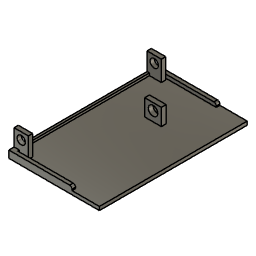
uselessbox-top-2 (Autodesk Fusion 360 design; units mm, degrees)
Autodesk Fusion 360 part; units mm, degrees
sketch "Sketch1" plane through (0, 0, 0) normal (0, 0, 1) x (1, 0, 0)
  line L0 (-25, 50) -> (13, 50)
  line L1 (13, 50) -> (13, -12)
  line L2 (13, -12) -> (-25, -12)
  line L3 (-25, -12) -> (-25, 50)
  line L4 (-25, 50) -> (-22.8, 50)
  line L5 (-22.8, 50) -> (-22.8, 47.8)
  line L6 (-22.8, 47.8) -> (-25, 47.8)
  line L7 (-25, 47.8) -> (-25, 50)
  line L8 (-25, 47.8) -> (-20, 47.8)
  line L9 (-20, 47.8) -> (-20, 47)
  line L10 (-20, 47) -> (-25, 47)
  line L11 (-25, 47) -> (-25, 47.8)
  line L12 (-25, -12) -> (-22.8, -12)
  line L13 (-22.8, -12) -> (-22.8, -9.8)
  line L14 (-22.8, -9.8) -> (-25, -9.8)
  line L15 (-25, -9.8) -> (-25, -12)
  line L16 (-25, -9.8) -> (-20, -9.8)
  line L17 (-20, -9.8) -> (-20, -9)
  line L18 (-20, -9) -> (-25, -9)
  line L19 (-25, -9) -> (-25, -9.8)
  line L20 (-25, -12) -> (3, -12)
  line L21 (3, -12) -> (3, -10.5)
  line L22 (3, -10.5) -> (-25, -10.5)
  line L23 (-25, -10.5) -> (-25, -12)
  line L24 (-25, 50) -> (3, 50)
  line L25 (3, 50) -> (3, 48.5)
  line L26 (3, 48.5) -> (-25, 48.5)
  line L27 (-25, 48.5) -> (-25, 50)
  dimension "d1" = 38
  dimension "d2" = 62
  dimension "d3" = 2.2
  dimension "d4" = 2.2
  dimension "d5" = 5
  dimension "d6" = 0.8
  dimension "d7" = 2.2
  dimension "d8" = 2.2
  dimension "d9" = 5
  dimension "d10" = 0.8
  dimension "d11" = 28
  dimension "d12" = 1.5
  dimension "d13" = 28
  dimension "d14" = 1.5
  constraint horizontal L0
  constraint vertical L1
  constraint horizontal L2
  constraint vertical L3
  constraint horizontal L4
  constraint vertical L5
  constraint horizontal L6
  constraint vertical L7
  constraint horizontal L8
  constraint vertical L9
  constraint horizontal L10
  constraint vertical L11
  constraint horizontal L12
  constraint vertical L13
  constraint horizontal L14
  constraint vertical L15
  constraint horizontal L16
  constraint vertical L17
  constraint horizontal L18
  constraint vertical L19
  constraint horizontal L20
  constraint vertical L21
  constraint horizontal L22
  constraint vertical L23
  constraint horizontal L24
  constraint vertical L25
  constraint horizontal L26
  constraint vertical L27
  measures "d1" distance of L0.start L0.end
  measures "d2" distance of L0.start L2.end
  measures "d3" distance of L0.start L4.end
  measures "d4" distance of L0.start L6.end
  measures "d5" distance of L6.end L8.end
  measures "d6" distance of L6.end L10.end
  measures "d7" distance of L2.end L12.end
  measures "d8" distance of L2.end L14.end
  measures "d9" distance of L14.end L16.end
  measures "d10" distance of L14.end L18.end
  measures "d11" distance of L2.end L20.end
  measures "d12" distance of L2.end L22.end
  measures "d13" distance of L0.start L24.end
  measures "d14" distance of L0.start L26.end
extrude "Extrude1" add sketch "Sketch1" along normal blind 6 contours L3 L6 L8 L9 L10 L11 | L3 L14 L16 L17 L18 L19 makes body 1 at (-21.6667, 47.8, 2) makes body 2 at (-21.6667, -9, 2)
extrude "Extrude3" add sketch "Sketch1" against normal blind 1.5 separate body makes body 3
sketch "Sketch2" plane through (0, 0, 0) normal (0, 0, 1) x (1, 0, 0)
  line L0 (-10, 32) -> (-3, 32)
  line L1 (-3, 32) -> (-3, 30)
  line L2 (-3, 30) -> (-10, 30)
  line L3 (-10, 30) -> (-10, 32)
  constraint horizontal L0
  constraint vertical L1
  constraint horizontal L2
  constraint vertical L3
extrude "Extrude4" add sketch "Sketch2" along normal blind 6 bodies 3
sketch "Sketch3" plane through (0, 30, 0) normal (0, -1, 0) x (1, 0, 0)
  line L0 (-10, 0) -> (-3, 0)
  line L1 (-3, 0) -> (-3, 6)
  line L2 (-3, 6) -> (-10, 6)
  line L3 (-10, 6) -> (-10, 0)
  circle A0 centre (-6.5, 3) radius 2
extrude "Extrude5" cut sketch "Sketch3" against normal blind 2 contours A0 bodies 3
sketch "Sketch4" plane through (0, -9.8, 0) normal (0, -1, 0) x (1, 0, 0)
  line L0 (-25, 0) -> (-20, 0)
  line L1 (-20, 0) -> (-20, 6)
  line L2 (-20, 6) -> (-25, 6)
  line L3 (-25, 6) -> (-25, 0)
  line L4 (-25, 0) -> (-22, 0)
  line L5 (-22, 0) -> (-22, 4.5)
  line L6 (-22, 4.5) -> (-25, 4.5)
  line L7 (-25, 4.5) -> (-25, 0)
  circle A0 centre (-22, 4.5) radius 1.75
  dimension "d25" = 3
  dimension "d26" = 4.5
  dimension "d27" = 3.5
  constraint horizontal L4
  constraint vertical L5
  constraint horizontal L6
  constraint vertical L7
  constraint coincident L0.start L3.end
  constraint coincident L5.end L6.start
  measures "d25" distance of L0.start L4.end
  measures "d26" distance of L0.start L6.end
  measures "d27" diameter of A0
extrude "Extrude6" add 2 faces at (-23.3333, -9.5333, 6) (-23.3333, 47.5333, 6) along direction (0, 0, 1) blind 1.5 on bodies 1 2 bodies 2 1 3
extrude "Extrude7" add 2 faces at (-20, -9.5333, 2.5) (-20, 47.5333, 2.5) along direction (1, 0, 0) blind 1 on bodies 1 2 bodies 1 2 3
extrude "Extrude8" cut sketch "Sketch4" against normal blind 60 contours L5 L6 A0 | L2 L5 L6 A0 | L2 A0 bodies 1
extrude "Extrude10" add 1 faces at (-12.3333, 29.3333, -1.5) along direction (0, 0, -1) blind 2 on bodies 1 bodies 1
extrude "Extrude11" cut sketch "Sketch1" against normal blind 1 contours L0 L1 L2 L3 L5 L8 L9 L10 L13 L16 L17 L18 L21 L22 L25 L26 bodies 1 makes body 4 at (-9.5, 32, 3)
extrude "Extrude12" cut 2 faces at (3, -11.5, -0.3333) (3, 49.5, -0.3333) along direction (-1, 0, 0) blind 1 on bodies 1 bodies 1
extrude "Extrude13" add 1 faces at (-20, 47.5333, -0.3333) along direction (1, 0, 0) blind 1 on bodies 1 bodies 1
extrude "Extrude14" add 1 faces at (-20, -9.5333, -0.3333) along direction (1, 0, 0) blind 1 on bodies 1 bodies 1
extrude "Extrude15" add 1 faces at (-7.6667, 31.3333, 0) along direction (0, 0, -1) blind 1 on bodies 4 bodies 1 4
extrude "Extrude16" cut 1 faces at (-12.3333, 29.3333, -3.5) along direction (0, 0, 1) blind 1 on bodies 1 bodies 1
extrude "Extrude18" add 2 faces at (-15.2667, 49.5, 0) (-15.2667, -11.5, 0) along direction (0, 0, 1) blind 0.5 on bodies 1 bodies 1
sketch "Sketch5" plane through (0, 0, -1) normal (0, 0, 1) x (-1, 0, 0)
  line L0 (3, -30) -> (10, -30)
  line L1 (10, -30) -> (10, -32)
  line L2 (10, -32) -> (3, -32)
  line L3 (3, -32) -> (3, -30)
  line L4 (25, 9) -> (19, 9)
  line L5 (19, 9) -> (19, 9.8)
  line L6 (19, 9.8) -> (22.8, 9.8)
  line L7 (22.8, 9.8) -> (22.8, 10.5)
  line L8 (22.8, 10.5) -> (-2, 10.5)
  line L9 (-2, 10.5) -> (-2, 12)
  line L10 (-2, 12) -> (-13, 12)
  line L11 (-13, 12) -> (-13, -50)
  line L12 (-13, -50) -> (-2, -50)
  line L13 (-2, -50) -> (-2, -48.5)
  line L14 (-2, -48.5) -> (22.8, -48.5)
  line L15 (22.8, -48.5) -> (22.8, -47.8)
  line L16 (22.8, -47.8) -> (19, -47.8)
  line L17 (19, -47.8) -> (19, -47)
  line L18 (19, -47) -> (25, -47)
  line L19 (25, -47) -> (25, 9)
  line L20 (25, 9) -> (24, 9)
  line L21 (24, 9) -> (24, -47)
  line L22 (24, -47) -> (25, -47)
  line L23 (25, -47) -> (25, 9)
  constraint horizontal L20
  constraint vertical L21
  constraint horizontal L22
  constraint vertical L23
  constraint coincident L18 L21.end
  constraint coincident L4.start L19.end
extrude "Extrude19" add sketch "Sketch5" along normal blind 1 contours L4 L18 L19 L20 L21 L22 L23 bodies 1
extrude "Extrude20" add 1 faces at (-21.6231, -9, 0.585) along direction (0, 1, 0) blind 0.5 on bodies 1 bodies 1
extrude "Extrude21" add 1 faces at (-21.6231, 47, 0.585) along direction (0, -1, 0) blind 0.5 on bodies 1 bodies 1
extrude "Extrude22" cut 2 faces at (2, 49, -0.5) (2, -11.5, 0) along direction (-1, 0, 0) blind 0.5 on bodies 1 bodies 1
fillet "Fillet3" radius 1 2 edges at (1.5, -11.25, 0.5) (1.5, 49.25, 0.5) on bodies 1
extrude "Extrude23" add 1 faces at (-21.6231, 46.5, 0.585) along direction (0, -1, 0) blind 0.5 on bodies 1 bodies 1
extrude "Extrude24" add 1 faces at (-21.6231, -8.5, 0.585) along direction (0, 1, 0) blind 0.5 on bodies 1 bodies 1
